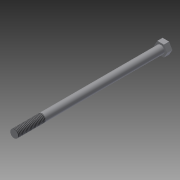
# Autodesk Inventor part: 7in bolt
Saved by Autodesk Inventor 2014 SP1 (Build 180222100, 222)
## iProperties
Created: 2013-12-17
Part Number: 7in bolt
Material: Generic
Document SubType Name: Modeling
Designer: habib asif
Density: 1 g/cm^3
Appearance: Default
Author: habib asif
Autodesk Inventor part; units mm, degrees
ref_plane "YZ Plane" through (0, 0, 0) normal (1, 0, 0) x (0, 1, 0)
ref_plane "XZ Plane" through (0, 0, 0) normal (0, 1, 0) x (-1, 0, 0)
ref_plane "XY Plane" through (0, 0, 0) normal (0, 0, 1) x (1, 0, 0)
sketch "Sketch1" plane through (0, 0, 0) normal (0, 0, 1) x (1, 0, 0)
  line L0 (-3.9687, 6.8741) -> (3.9687, 6.8741)
  line L1 (3.9687, 6.8741) -> (7.9375, 0)
  line L2 (7.9375, 0) -> (3.9687, -6.8741)
  line L3 (3.9687, -6.8741) -> (-3.9688, -6.8741)
  line L4 (-3.9688, -6.8741) -> (-7.9375, 0)
  line L5 (-7.9375, 0) -> (-3.9687, 6.8741)
  point P0 (0, 0)
  point P1 (0, 6.8741)
  dimension "d0" = 15.875
  constraints: 12 end point, 1 midpoint, 1 vertical alignment, 13 other
  measures "d0" distance of L1.end L4.end
extrude "Extrusion1" add sketch "Sketch1" along normal blind 6.35
sketch "Sketch2" plane through (0, 0, 6.35) normal (0, 0, 1) x (1, 0, 0)
  circle A0 centre (0, 0) radius 4.7625
  dimension "d3" = 9.525
  constraints: 1 centre point
  measures "d3" diameter of A0
extrude "Extrusion2" add sketch "Sketch2" along normal blind 177.8
thread "Thread1" size "3/8-16 UNC" class "2A" standard "ANSI Unified Screw Threads" length 33.655
body "Solid1"
